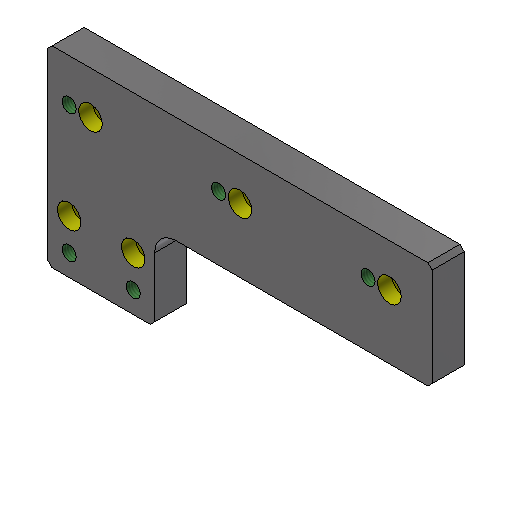
# Autodesk Inventor part: TL20240901-10320CV-016
Saved by Autodesk Inventor 2022.5 (Build 265521000, 521)
## iProperties
Category: FOLLOWER UNIT ASSY
Company: 현대 트랜시스
RuleStatus: InUse
Created: 2023-04-10
Part Number: TL20240901-10320CV-016
Checked By: 김형민
Engr Approved By: 김형민
User Status: 1/1 x6
Material: SS400
Description: 0
Document SubType Name: Modeling
Mfg Approved By: 호상태
Designer: 박성규
Stock Number: 016
Density: 7.85 g/cm^3
Appearance: Plating Zinc White
Project: MEa-PJT 2LINE
BeforeDocSave0: file://Part Design STD iLogic
DETAIL: Coveryor Assembly
M/C TITLE: CJ 제일제당 협동로봇 포장시스탬 PILOT 장비
PARTS NAME: Bracket
SPECIFICATION: TA20221101-CV200000-015
DocNumber: 221118_Standard_v1
Folder: .\
VDS_Category: 엔지니어링
Detail Description: Processed products
Title: BLOCK
Subject: MEa차종 시트조립2라인
Author: 박성규
Revision Number: A
Autodesk Inventor part; units mm, degrees
ref_plane "YZ Plane" through (0, 0, 0) normal (1, 0, 0) x (0, 1, 0)
ref_plane "XZ Plane" through (0, 0, 0) normal (0, 1, 0) x (-1, 0, 0)
ref_plane "XY Plane" through (0, 0, 0) normal (0, 0, 1) x (1, 0, 0)
sketch "스케치9" plane through (0, 0, 0) normal (0, 0, 1) x (1, 0, 0)
  line L0 (-90, 45) -> (90, 45)
  line L1 (90, 45) -> (90, -45)
  line L2 (90, -45) -> (-90, -45)
  line L3 (-90, -45) -> (-90, 45)
  line L4 (-90, 45) -> (90, -45) construction
  line L5 (90, 45) -> (-90, -45) construction
  line L6 (90, -45) -> (-40, -45)
  line L7 (-40, -45) -> (-40, -5)
  line L8 (-40, -5) -> (90, -5)
  line L9 (90, -5) -> (90, -45)
  point P0 (0, 0)
  point P1 (-40, -45)
  dimension "d40" = 180
  dimension "d41" = 90
  dimension "d44" = 130
  dimension "d45" = 40
  constraints: 20 end point, 4 parallel, 2 horizontal, 2 midpoint, 2 perpendicular
  measures "d40" distance of L0.start L0.end
  measures "d41" distance of L0.end L1.end
  measures "d44" distance of L7.end L8.end
  measures "d45" distance between parallel lines of L6 L8
extrude "돌출5" add sketch "스케치9" along normal blind 15 contours L0 L1 L8 L7 L2 L3
fillet "모깎기2" radius 10 1 edges at (-40, -5, 7.5)
chamfer "모따기1" distance 2 angle 45 5 edges at (-40, -45, 7.5) (-90, -45, 7.5) (-90, 45, 7.5) (90, 45, 7.5) (90, -5, 7.5)
sketch "스케치10" plane through (0, 0, 15) normal (0, 0, 1) x (1, 0, 0)
  line L0 (-90, 43) -> (-90, -43) construction
  line L1 (-88, -45) -> (-42, -45) construction
  point P0 (0, 0)
  point P1 (-80, -20)
  point P2 (-50, -20)
  point P3 (-70, 25)
  point P4 (0, 25)
  point P5 (70, 25)
  dimension "d52" = 25
  dimension "d53" = 10
  dimension "d54" = 70
  dimension "d55" = 70
  dimension "d56" = 70
  dimension "d77" = 30
  dimension "d79" = 20
  constraints: 3 horizontal alignment
  measures "d52" distance from line of point (-50, -20) L1
  measures "d53" distance from line of L0 point (-80, -20)
  measures "d54" distance from line of point (-70, 25) L1
  measures "d55" distance of point (0, 25) point (-70, 25)
  measures "d56" distance of point (70, 25) point (0, 25)
  measures "d77" distance of point (-80, -20) point (-50, -20)
  measures "d79" distance from line of L0 point (-70, 25)
hole "구멍3" at (-80, -20, 15) at (-50, -20, 15) at (-70, 25, 15) at (0, 25, 15) at (70, 25, 15) direction (0, 0, -1) diameter 6.6 end through all counterbore diameter 11 counterbore depth 6.5 clearance for "Socket Head Cap Screw" size "M6" standard "TS Profile"
sketch "스케치11" plane through (0, 0, 15) normal (0, 0, 1) x (1, 0, 0)
  line L0 (-90, 43) -> (-90, -43) construction
  line L1 (-88, -45) -> (-42, -45) construction
  point P0 (0, 0)
  point P1 (-80, -35)
  point P2 (-80, 25)
  point P3 (-10, 25)
  point P4 (-50, -35)
  point P5 (60, 25)
  dimension "d64" = 10
  dimension "d65" = 10
  dimension "d66" = 70
  dimension "d67" = 30
  dimension "d68" = 70
  dimension "d69" = 70
  dimension "d78" = 10
  constraints: 3 horizontal alignment
  measures "d64" distance from line of point (-80, -35) L0
  measures "d65" distance from line of point (-80, -35) L1
  measures "d66" distance from line of point (-80, 25) L1
  measures "d67" distance of point (-50, -35) point (-80, -35)
  measures "d68" distance of point (-10, 25) point (-80, 25)
  measures "d69" distance of point (60, 25) point (-10, 25)
  measures "d78" distance from line of L0 point (-80, 25)
hole "구멍4" at (-80, -35, 15) at (-80, 25, 15) at (-10, 25, 15) at (-50, -35, 15) at (60, 25, 15) direction (0, 0, -1) diameter 6.647 end through all thread size "M8x1.25" class "6H" standard "TS profile"
equation "\"d56\" = d55"
equation "\"d69\" = d68"
